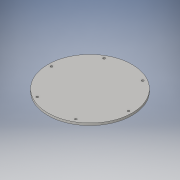
# Autodesk Inventor part: Acrylic lense
Saved by Autodesk Inventor 2016 (Build 200138000, 138)
## iProperties
Created: 2017-09-28
Part Number: Acrylic lense
Material: Generic
Document SubType Name: Modeling
Designer: Student
Density: 1 g/cm^3
Appearance: Default
Author: Student
Autodesk Inventor part; units mm, degrees
ref_plane "YZ Plane" through (0, 0, 0) normal (1, 0, 0) x (0, 1, 0)
ref_plane "XZ Plane" through (0, 0, 0) normal (0, 1, 0) x (-1, 0, 0)
ref_plane "XY Plane" through (0, 0, 0) normal (0, 0, 1) x (1, 0, 0)
sketch "Sketch2" plane through (0, 0, 0) normal (0, 1, 0) x (-1, 0, 0)
  circle A0 centre (0, 0) radius 60.198
  dimension "d3" = 120.396
  constraints: 1 centre point, 1 coincident
  measures "d3" diameter of A0
extrude "Extrusion1" add sketch "Sketch2" along normal blind 3.175
sketch "Sketch3" plane through (0, 3.175, 0) normal (0, 1, 0) x (1, 0, 0)
  point P0 (0, 0)
  point P1 (-55.245, 0)
  point P2 (-27.6225, -47.8436)
  point P3 (27.6225, -47.8436)
  point P4 (55.245, 0)
  point P5 (27.6225, 47.8436)
  point P6 (-27.6225, 47.8436)
  dimension "d6" = 55.245
  dimension "d9" = 360
  constraints: 7 other
  measures "d6" distance of point (0, 0) point (-55.245, 0)
hole "Hole1" at (-55.245, 3.175, 0) at (-27.6225, 3.175, 47.8436) at (27.6225, 3.175, 47.8436) at (55.245, 3.175, 0) at (27.6225, 3.175, -47.8436) at (-27.6225, 3.175, -47.8436) direction (0, -1, 0) diameter 3 depth 25.4 tip angle 118
body "Solid1"
